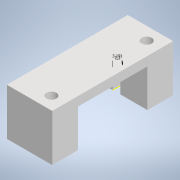
# Autodesk Inventor part: держалка_серво_бровь_нижняя
Saved by Autodesk Inventor 2020 (Build 240168000, 168)
## iProperties
Created: 2022-03-02
Part Number: держалка_серво_бровь_нижняя
Material: Типовые
Document SubType Name: Modeling
Designer: Администратор
Density: 1 g/cm^3
Appearance: По умолчанию
Author: Администратор
Autodesk Inventor part; units mm, degrees
ref_plane "YZ Plane" through (0, 0, 0) normal (1, 0, 0) x (0, 1, 0)
ref_plane "XZ Plane" through (0, 0, 0) normal (0, 1, 0) x (-1, 0, 0)
ref_plane "XY Plane" through (0, 0, 0) normal (0, 0, 1) x (1, 0, 0)
sketch "Эскиз1" plane through (0, 0, 0) normal (0, 1, 0) x (-1, 0, 0)
  line L0 (0, 0) -> (-10.5018, 0)
  line L1 (0, 0) -> (15, 0)
  line L2 (15, 0) -> (15, -20)
  line L3 (15, -20) -> (0, -20)
  line L4 (0, -20) -> (0, 0)
  line L5 (15, 0) -> (15, 20)
  line L6 (15, 20) -> (0, 20)
  line L7 (0, 20) -> (0, 0)
  dimension "d5" = 15
  dimension "d6" = 20
  constraints: 16 end point, 2 horizontal, 2 parallel, 2 symmetric about line, 1 perpendicular
  measures "d5" distance of L2.end L3.end
  measures "d6" distance of L1.end L2.end
extrude "Выдавливание1" add sketch "Эскиз1" along normal blind 3
sketch "Эскиз3" plane through (0, 0, 0) normal (0, -1, 0) x (1, 0, 0)
  line L0 (-15, 20) -> (0, 20) projected
  line L1 (-9, 16.5) -> (-11.5, 16.5)
  line L2 (-11.5, 16.5) -> (-11.5, 11.5)
  line L3 (-9, 11.5) -> (-9, 16.5)
  line L4 (0, 0) -> (-5.7861, 0)
  line L5 (-9, -16.5) -> (-11.5, -16.5)
  line L6 (-11.5, -16.5) -> (-11.5, -11.5)
  line L7 (-9, -11.5) -> (-9, -16.5)
  line L8 (-9, -11.5) -> (0, -11.5)
  line L9 (0, 20) -> (0, -20) projected
  line L10 (0, -20) -> (-15, -20) projected
  line L11 (0, -20) -> (-15, -20)
  line L12 (-15, -20) -> (-15, -11.5)
  line L13 (-15, -20) -> (-15, 20) projected
  line L14 (-11.5, -11.5) -> (-15, -11.5)
  line L15 (0, -11.5) -> (0, -20)
  line L16 (-11.5, 16.5) -> (-11.5, 11.5)
  line L17 (-9, 11.5) -> (-9, 16.5)
  line L18 (-9, 16.5) -> (-11.5, 16.5)
  line L19 (-9, 11.5) -> (0, 11.5)
  line L20 (0, 20) -> (-15, 20)
  line L21 (0, 20) -> (-15, 20)
  line L22 (-15, 20) -> (-15, 11.5)
  line L23 (-11.5, 11.5) -> (-15, 11.5)
  line L24 (0, 11.5) -> (0, 20)
  point P0 (-15, 11.5)
  constraints: 42 end point, 6 symmetric about line, 4 point on line, 3 horizontal, 2 equal length, 2 perpendicular, 1 vertical
extrude "Выдавливание2" add sketch "Эскиз3" along normal blind 12.5 contours L0 L9 L19 L3 L1 L2 L23 L13 | L14 L6 L5 L7 L8 L9 L10 L12
sketch "Эскиз4" plane through (0, -12.5, 0) normal (0, -1, 0) x (1, 0, 0)
  line L0 (-15, 20) -> (0, 20) projected
  line L1 (0, 20) -> (-4.5, 20)
  circle A0 centre (-4.5, 15.75) radius 1.65
  line L2 (0, 0) -> (-4.5, 0)
  circle A1 centre (-4.5, -15.75) radius 1.65
  dimension "d18" = 3.3
  constraints: 4 end point, 2 centre point, 1 horizontal, 1 point on line, 1 symmetric about line, 1 other
  measures "d18" diameter of A0
extrude "Выдавливание3" cut sketch "Эскиз4" against normal through all
sketch "Эскиз5" plane through (-11.5, 0, -11.5) normal (1, 0, 0) x (0, 0, -1)
  line L0 (0, -12.5) -> (8.5, -12.5) projected
  line L1 (4.25, -12.5) -> (4.25, -6)
  line L2 (0, -6) -> (3.191, -6)
  circle A0 centre (3.191, -6) radius 1.1
  line L3 (-11.5, 0) -> (-11.5, -8.8463)
  circle A1 centre (-26.191, -6) radius 1.1
  dimension "d20" = 3.191
  dimension "d21" = 2.2
  constraints: 6 end point, 2 centre point, 2 vertical, 1 coincident, 1 horizontal, 1 midpoint, 1 symmetric about line, 1 other
  measures "d20" distance of L2.start L2.end
  measures "d21" diameter of A0
